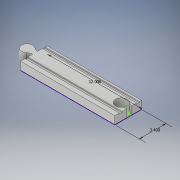
# Autodesk Inventor part: train track
Saved by Autodesk Inventor 2017 (Build 210142000, 142)
## iProperties
Created: 2017-04-27
Part Number: train track
Material: Generic
Document SubType Name: Modeling
Designer: 167942
Density: 1 g/cm^3
Appearance: Default
Author: 167942
Autodesk Inventor part; units mm, degrees
ref_plane "YZ Plane" through (0, 0, 0) normal (1, 0, 0) x (0, 1, 0)
ref_plane "XZ Plane" through (0, 0, 0) normal (0, 1, 0) x (-1, 0, 0)
ref_plane "XY Plane" through (0, 0, 0) normal (0, 0, 1) x (1, 0, 0)
sketch "Sketch1" plane through (0, 0, 0) normal (0, 1, 0) x (-1, 0, 0)
  line L0 (0, 0) -> (304.8, 0)
  line L1 (304.8, 0) -> (304.8, -86.36)
  line L2 (304.8, -86.36) -> (0, -86.36)
  line L3 (0, -86.36) -> (0, 0)
  circle A0 centre (25.4, -47.2363) radius 19.05
  circle A1 centre (330.2, -47.2363) radius 17.78
  line L4 (34.5288, -55.4913) -> (0, -55.4913)
  line L5 (34.5288, -38.9813) -> (0, -38.9813)
  line L6 (34.5288, -38.9813) -> (34.5288, -55.4913)
  line L7 (0, -38.9813) -> (0, -55.4913)
  line L8 (331.681, -55.4913) -> (282.1836, -55.4913)
  line L9 (331.681, -38.9813) -> (282.1836, -38.9813)
  line L10 (331.681, -38.9813) -> (331.681, -55.4913)
  line L11 (282.1836, -38.9813) -> (282.1836, -55.4913)
  dimension "d0" = 304.8
  dimension "d1" = 86.36
  constraints: 24 end point, 3 horizontal, 3 parallel, 2 centre point, 2 point on line, 2 vertical, 1 collinear, 1 perpendicular
  measures "d0" distance of L1.end L2.end
  measures "d1" distance of L2.end L0.start
extrude "Extrusion1" add sketch "Sketch1" along normal blind 25.4
extrude "Extrusion2" cut sketch "Sketch1" along normal blind 25.4 contours L5 A0 L4 L3 | L5 L6 L4 A0 | A0 L4 L6 L5
fillet "Fillet1" radius 22.86 4 edges at (-8.2315, 12.7, -55.4913) (-8.2315, 12.7, -38.9813) (-314.4525, 12.7, -38.9813) (-314.4525, 12.7, -55.4913)
sketch "Sketch2" plane through (0, 0, 0) normal (1, 0, 0) x (0, 0, -1)
  line L0 (38.9813, 25.4) -> (0, 25.4) projected
  line L1 (14.8709, 25.4) -> (23.7033, 25.4)
  line L2 (23.7033, 25.4) -> (23.7033, 22.0925)
  line L3 (23.7033, 22.0925) -> (14.8709, 22.0925)
  line L4 (14.8709, 22.0925) -> (14.8709, 25.4)
  line L5 (86.36, 25.4) -> (55.4913, 25.4) projected
  line L6 (70.9256, 25.4) -> (79.3317, 25.4)
  line L7 (79.3317, 25.4) -> (79.3317, 22.0925)
  line L8 (79.3317, 22.0925) -> (70.9256, 22.0925)
  line L9 (70.9256, 22.0925) -> (70.9256, 25.4)
  point P0 (0, 0)
  constraints: 16 end point, 4 parallel, 2 horizontal, 2 perpendicular, 2 point on line, 1 midpoint
extrude "Extrusion3" cut sketch "Sketch2" against normal blind 379.4125
body "Solid1"
